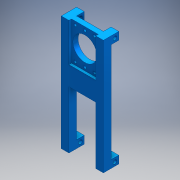
# Autodesk Inventor part: framesideRight
Saved by Autodesk Inventor 2016 (Build 200138000, 138)
## iProperties
Created: 2016-05-18
Part Number: framesideRight
Material: ABS Plastic
Document SubType Name: Modeling
Designer: hesaon
Density: 1.06 g/cm^3
Appearance: Smooth - White
Author: hesaon
Autodesk Inventor part; units mm, degrees
ref_plane "YZ Plane" through (0, 0, 0) normal (1, 0, 0) x (0, 1, 0)
ref_plane "XZ Plane" through (0, 0, 0) normal (0, 1, 0) x (-1, 0, 0)
ref_plane "XY Plane" through (0, 0, 0) normal (0, 0, 1) x (1, 0, 0)
sketch "Sketch1" plane through (0, 0, 0) normal (0, 1, 0) x (-1, 0, 0)
  line L0 (66, 0) -> (66, -180)
  line L1 (66, -180) -> (0, -180)
  line L2 (0, -180) -> (0, 0)
  line L3 (12, -168) -> (54, -168)
  line L4 (54, -60) -> (12, -60)
  line L5 (54, -90) -> (12, -90)
  line L6 (54, -168) -> (54, -90)
  line L7 (12, -90) -> (12, -168)
  line L8 (0, 0) -> (12, 0)
  line L9 (54, 0) -> (66, 0)
  line L10 (12, -60) -> (12, 0)
  line L11 (54, -60) -> (54, 0)
  dimension "d0" = 66
  dimension "d3" = 42
  dimension "d4" = 12
  dimension "d5" = 12
  dimension "d7" = 30
  dimension "d165" = 12
  dimension "d166" = 60
  dimension "d167" = 12
  dimension "d168" = 78
  dimension "d169" = 42
  dimension "d170" = 60
  dimension "d171" = 30
  dimension "d172" = 78
  dimension "d173" = 12
  constraints: 24 end point, 3 parallel, 2 horizontal, 2 perpendicular, 1 vertical
  measures "d0" distance of L0.end L1.end
  measures "d3" distance of L3.start L3.end
  measures "d4" distance from line of L1 L3.start
  measures "d5" distance from line of L0 L3.end
  measures "d7" distance of L5.end L4.end
  measures "d165" distance of L8.end L2.end
  measures "d166" distance of L8.end L4.end
  measures "d167" distance of L0.start L9.start
  measures "d168" distance of L3.start L5.end
  measures "d169" distance of L4.start L4.end
  measures "d170" distance of L9.start L4.start
  measures "d171" distance of L5.start L4.start
  measures "d172" distance of L3.end L5.start
  measures "d173" horizontal distance of L3.end L0.end
extrude "Extrusion1" add sketch "Sketch1" along normal blind 12
sketch "Sketch6" plane through (0, 0, 0) normal (0, -1, 0) x (1, 0, 0)
  line L0 (-54, -90) -> (-54, -168) projected
  line L1 (-54, -168) -> (-12, -168)
  line L2 (-12, -168) -> (-12, -180)
  line L3 (-12, -180) -> (-54, -180)
  line L4 (-54, -180) -> (-54, -168)
  point P0 (0, 0)
  dimension "d100" = 42
  dimension "d101" = 12
  constraints: 8 end point, 2 parallel, 1 horizontal, 1 perpendicular
  measures "d100" distance of L2.end L3.end
  measures "d101" distance of L1.end L2.end
extrude "Extrusion7" cut sketch "Sketch6" against normal up to next
sketch "Sketch13" plane through (0, 12, 0) normal (0, 1, 0) x (1, 0, 0)
  line L0 (0, 180) -> (-12, 180) projected
  line L1 (0, 180) -> (-12, 180)
  line L2 (-12, 180) -> (-12, 168)
  line L3 (-12, 168) -> (0, 168)
  line L4 (0, 168) -> (0, 180)
  line L5 (-54, 180) -> (-66, 180) projected
  line L6 (-54, 180) -> (-66, 180)
  line L7 (-66, 180) -> (-66, 168)
  line L8 (-66, 168) -> (-54, 168)
  line L9 (-54, 168) -> (-54, 180)
  point P0 (0, 0)
  dimension "d136" = 12
  dimension "d137" = 12
  dimension "d138" = 12
  dimension "d139" = 12
  constraints: 16 end point, 4 parallel, 2 horizontal, 2 perpendicular
  measures "d136" distance of L3.end L2.end
  measures "d137" distance of L2.end L1.end
  measures "d138" distance of L8.end L7.end
  measures "d139" distance of L7.end L6.end
extrude "Extrusion13" add sketch "Sketch13" along normal blind 12
sketch "Sketch14" plane through (0, 0, 0) normal (1, 0, 0) x (0, 0, -1)
  circle A0 centre (174, 18) radius 3
  line L0 (168, 12) -> (168, 24) projected
  line L1 (168, 24) -> (180, 24) projected
  point P0 (0, 0)
  dimension "d142" = 6
  dimension "d143" = 6
  dimension "d144" = 6
  constraints: 1 centre point
  measures "d142" diameter of A0
  measures "d143" distance from line of L0 A0.centre
  measures "d144" distance from line of L1 A0.centre
extrude "Extrusion14" cut sketch "Sketch14" against normal blind 66
sketch "Sketch15" plane through (-12, 0, -90) normal (0, 0, -1) x (-1, 0, 0)
  circle A0 centre (7, 6) radius 3
  circle A1 centre (24, 6) radius 3
  line L0 (0, 0) -> (0, 24) projected
  line L1 (0, 12) -> (42, 12) projected
  point P0 (-12, 0)
  dimension "d147" = 6
  dimension "d148" = 6
  dimension "d149" = 7
  dimension "d150" = 17
  dimension "d151" = 6
  dimension "d152" = 6
  constraints: 2 centre point
  measures "d147" diameter of A0
  measures "d148" diameter of A1
  measures "d149" distance from line of L0 A0.centre
  measures "d150" distance of A1.centre A0.centre
  measures "d151" distance from line of L1 A0.centre
  measures "d152" distance from line of L1 A1.centre
extrude "Extrusion15" cut sketch "Sketch15" against normal blind 6
sketch "Sketch16" plane through (0, 0, 0) normal (0, -1, 0) x (1, 0, 0)
  line L0 (-54, -12) -> (-12, -12) projected
  line L1 (-12, -12) -> (-54, -12)
  line L2 (-54, -12) -> (-54, 0)
  line L3 (-54, 0) -> (-12, 0)
  line L4 (-12, 0) -> (-12, -12)
  point P0 (0, 0)
  constraints: 8 end point, 2 parallel, 1 horizontal, 1 perpendicular
extrude "Extrusion17" cut sketch "Sketch16" against normal blind 4
sketch "Sketch17" plane through (0, 12, 0) normal (0, 1, 0) x (1, 0, 0)
  line L0 (-54, 60) -> (-12, 60) projected
  line L1 (-66, 0) -> (-54, 0) projected
  line L2 (-12, 60) -> (-54, 60)
  line L3 (-54, 60) -> (-54, 0)
  line L4 (-54, 0) -> (-12, 0)
  line L5 (-12, 0) -> (-12, 60)
  circle A0 centre (-33, 30) radius 18.75
  circle A1 centre (-33, 5) radius 2.1
  circle A2 centre (-48, 5) radius 2.1
  circle A3 centre (-18, 5) radius 2.1
  line L6 (-12, 0) -> (0, 0) projected
  circle A4 centre (-18, 55) radius 2.1
  circle A5 centre (-33, 55) radius 2.1
  circle A6 centre (-48, 55) radius 2.1
  dimension "d174" = 37.5
  dimension "d175" = 21
  dimension "d176" = 30
  dimension "d177" = 4.2
  dimension "d178" = 4.2
  dimension "d179" = 4.2
  dimension "d180" = 21
  dimension "d181" = 15
  dimension "d182" = 15
  dimension "d183" = 5
  dimension "d184" = 5
  dimension "d185" = 5
  dimension "d186" = 4.2
  dimension "d187" = 4.2
  dimension "d188" = 4.2
  dimension "d189" = 5
  dimension "d190" = 5
  dimension "d191" = 5
  dimension "d192" = 15
  dimension "d193" = 15
  dimension "d194" = 21
  constraints: 8 end point, 7 centre point, 2 parallel, 1 horizontal, 1 perpendicular
  measures "d174" diameter of A0
  measures "d175" horizontal distance of L4.end A0.centre
  measures "d176" vertical distance of L1.end A0.centre
  measures "d177" diameter of A1
  measures "d178" diameter of A2
  measures "d179" diameter of A3
  measures "d180" horizontal distance of L4.end A1.centre
  measures "d181" distance of A1.centre A3.centre
  measures "d182" distance of A2.centre A1.centre
  measures "d183" distance from line of L6 A3.centre
  measures "d184" distance from line of L6 A1.centre
  measures "d185" distance from line of L6 A2.centre
  measures "d186" diameter of A4
  measures "d187" diameter of A5
  measures "d188" diameter of A6
  measures "d189" distance from line of L2 A4.centre
  measures "d190" distance from line of L0 A5.centre
  measures "d191" distance from line of L0 A6.centre
  measures "d192" distance of A5.centre A4.centre
  measures "d193" distance of A6.centre A5.centre
  measures "d194" distance from line of L5 A5.centre
extrude "Extrusion19" add sketch "Sketch17" against normal blind 8
sketch "Sketch18" plane through (0, 12, 0) normal (0, 1, 0) x (1, 0, 0)
  line L0 (0, 0) -> (0, 168) projected
  line L1 (0, 0) -> (-12, 0)
  line L2 (-12, 0) -> (-12, 12)
  line L3 (-12, 12) -> (0, 12)
  line L4 (0, 12) -> (0, 0)
  line L5 (-66, 168) -> (-66, 0) projected
  line L6 (-66, 0) -> (-54, 0)
  line L7 (-54, 0) -> (-54, 12)
  line L8 (-54, 12) -> (-66, 12)
  line L9 (-66, 12) -> (-66, 0)
  dimension "d197" = 12
  dimension "d198" = 12
  dimension "d199" = 12
  dimension "d200" = 12
  constraints: 16 end point, 4 parallel, 2 horizontal, 2 perpendicular
  measures "d197" distance of L2.end L3.end
  measures "d198" distance of L1.end L2.end
  measures "d199" distance of L8.end L7.end
  measures "d200" distance of L7.end L6.end
extrude "Extrusion20" add sketch "Sketch18" along normal blind 12
sketch "Sketch19" plane through (-66, 0, -180) normal (-1, 0, 0) x (0, 0, 1)
  circle A0 centre (174, 18) radius 3
  line L0 (168, 24) -> (180, 24) projected
  line L1 (168, 12) -> (168, 24) projected
  point P0 (180, 0)
  dimension "d203" = 6
  dimension "d204" = 6
  dimension "d205" = 6
  constraints: 1 centre point
  measures "d203" diameter of A0
  measures "d204" distance from line of L0 A0.centre
  measures "d205" distance from line of L1 A0.centre
extrude "Extrusion21" cut sketch "Sketch19" against normal blind 66
body "Solid1"
